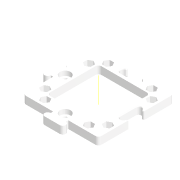
# Autodesk Inventor part: 10_Base_puzzle_v3
Saved by Autodesk Inventor 2022 (Build 260153000, 153)
## iProperties
Created: 2017-06-20
Part Number: 10_Base_puzzle_v3
Material: Generisch
Document SubType Name: Modeling
Designer: diederichbenedict
Density: 1 g/cm^3
Appearance: Weiß
Mass: 5.4697 g
Surface Area: 48.9743 cm^2
Volume: 5.4697 cm^3
Catalog Web Link: isInjectionmolded
Vendor: openUC2
d_part: 50,000 mm
d_o: 40,000 mm
d_i: 40,000 mm
Author: diederichbenedict
Autodesk Inventor part; units mm, degrees
ref_plane "YZ Plane" through (0, 0, 0) normal (1, 0, 0) x (0, 1, 0)
ref_plane "XZ Plane" through (0, 0, 0) normal (0, 1, 0) x (-1, 0, 0)
ref_plane "XY Plane" through (0, 0, 0) normal (0, 0, 1) x (1, 0, 0)
sketch "Skizze1" plane through (0, 0, 0) normal (0, 0, 1) x (1, 0, 0)
  line L0 (-17, 0) -> (-25, 0)
  line L1 (-25, 0) -> (-25, -23)
  line L2 (-23, -25) -> (0, -25)
  line L3 (0, -25) -> (0, -17)
  line L4 (-17, 0) -> (-17, -15)
  line L5 (-15, -17) -> (0, -17)
  arc A0 (-25, -23) -> (-23, -25) centre (-23, -23) ccw
  circle A1 centre (-20.8, -14.5) radius 2.55 construction
  circle A2 centre (-14.5, -20.8) radius 2.55 construction
  arc A3 (-17, -15) -> (-15, -17) centre (-15, -15) ccw
  circle A4 centre (-14.5, -20.8) radius 2.55 construction
  circle A5 centre (-20.8, -14.5) radius 2.55 construction
  line L6 (-30.497056, 0) -> (5.082843, 0) construction
  line L7 (0, -30.497056) -> (0, 5.082843) construction
  line L8 (-18.25, -13.027757) -> (-18.25, -15.972243)
  line L9 (-18.25, -15.972243) -> (-20.8, -17.444486)
  line L10 (-20.8, -17.444486) -> (-23.35, -15.972243)
  line L11 (-23.35, -15.972243) -> (-23.35, -13.027757)
  line L12 (-23.35, -13.027757) -> (-20.8, -11.555514)
  line L13 (-20.8, -11.555514) -> (-18.25, -13.027757)
  line L14 (-15.972243, -18.25) -> (-13.027757, -18.25)
  line L15 (-13.027757, -18.25) -> (-11.555514, -20.8)
  line L16 (-11.555514, -20.8) -> (-13.027757, -23.35)
  line L17 (-13.027757, -23.35) -> (-15.972243, -23.35)
  line L18 (-15.972243, -23.35) -> (-17.444486, -20.8)
  line L19 (-17.444486, -20.8) -> (-15.972243, -18.25)
  point P0 (-25, -25)
  point P1 (-17, -17)
  dimension "d278" = 25
  dimension "d279" = 25
  dimension "d2" = 8
  dimension "d281" = 8
  dimension "d282" = 2
  dimension "d286" = 5.1
  dimension "d_hole" = 5.1
  dimension "d290" = 20.8
  dimension "d" = 20.8
  dimension "d292" = 2
  dimension "d313" = 6.3
  dimension "d314" = 6.3
  dimension "d331" = 0
  dimension "d332" = 0
  constraints: 36 end point, 6 centre point, 6 tangent, 5 coincident, 4 parallel, 4 point on circle, 4 point on line, 2 collinear, 1 horizontal, 1 perpendicular, 26 other
  measures "d278" distance of L2.end point (-25, -25)
  measures "d279" distance of point (-25, -25) L0.end
  measures "d2" distance between parallel lines of L4 L1
  measures "d281" distance between parallel lines of L2 L5
  measures "d282" radius of A0
  measures "d286" diameter of A1
  measures "d_hole" diameter of A2
  measures "d290" distance from line of L0 A2.centre
  measures "d" distance from line of L3 A1.centre
  measures "d292" radius of A3
  measures "d313" horizontal distance of A1.centre A2.centre
  measures "d314" horizontal distance of A1.centre A2.centre
  measures "d331" radial gap between concentric circles of A2 A4
  measures "d332" radial gap between concentric circles of A1 A5
extrude "Extrusion1" add sketch "Skizze1" along normal blind 5
mirror "Mirror6" about plane through (-17, 0, 0) normal (0, 1, 0) of "Extrusion1"
mirror "Mirror7" about plane through (0, -25, 0) normal (1, 0, 0) of "Extrusion1", "Mirror6"
sketch "Sketch26" plane through (0, 0, 5) normal (0, 0, 1) x (1, 0, 0)
  line L0 (23, 25) -> (-23, 25)
  arc A0 (-23, 25) -> (-25, 23) centre (-23, 23) ccw
  line L1 (-25, -23) -> (-25, 23)
  arc A1 (-25, -23) -> (-23, -25) centre (-23, -23) ccw
  line L2 (-23, -25) -> (23, -25)
  arc A2 (23, -25) -> (25, -23) centre (23, -23) ccw
  line L3 (25, 23) -> (25, -23)
  arc A3 (25, 23) -> (23, 25) centre (23, 23) ccw
  line L4 (15, 17) -> (-15, 17)
  arc A4 (17, 15) -> (15, 17) centre (15, 15) ccw
  line L5 (17, 15) -> (17, -15)
  arc A5 (15, -17) -> (17, -15) centre (15, -15) ccw
  line L6 (-15, -17) -> (15, -17)
  arc A6 (-17, -15) -> (-15, -17) centre (-15, -15) ccw
  line L7 (-17, -15) -> (-17, 15)
  arc A7 (-15, 17) -> (-17, 15) centre (-15, 15) ccw
  line L8 (-25, -23) -> (-25, 23)
  line L9 (-28.6, -7) -> (-28.6, -7)
  line L10 (-30.6, -5) -> (-30.6, 5)
  line L11 (-28.6, 7) -> (-28.6, 7)
  line L12 (-25, 16.831111) -> (-25, -7)
  line L13 (-26.363932, 5) -> (-25, 5)
  line L14 (-25, -5) -> (-26.363932, -5)
  arc A8 (-30.6, -5) -> (-28.6, -7) centre (-28.6, -5) ccw
  arc A9 (-28.6, -7) -> (-26.612384, -5.222222) centre (-28.6, -5) ccw
  arc A10 (-28.6, 7) -> (-30.6, 5) centre (-28.6, 5) ccw
  arc A11 (-26.612384, 5.222222) -> (-28.6, 7) centre (-28.6, 5) ccw
  arc A12 (-26.363932, -5) -> (-26.612384, -5.222222) centre (-26.363932, -5.25) ccw
  arc A13 (-26.612384, 5.222222) -> (-26.363932, 5) centre (-26.363932, 5.25) ccw
  line L15 (-42.419899, 0) -> (36.719899, 0)
  point P0 (0, 0)
  point P1 (-24.031265, 1.861044)
  point P2 (-28.6, -7)
  point P3 (-25, -5)
  point P4 (-25, 5)
  point P5 (-28.6, 7)
  dimension "d293" = 5.6
  dimension "d300" = 2
  dimension "d301" = 0.25
  dimension "d365" = 7
  dimension "d367" = 7
  dimension "d385" = 5
  dimension "d386" = 5
  constraints: 12 end point, 12 point on circle, 10 tangent, 6 centre point, 4 equal radius, 3 parallel, 2 coincident, 2 point on line, 1 horizontal, 1 perpendicular, 1 other
  measures "d293" distance between parallel lines of L1 L10
  measures "d300" radius of A8
  measures "d301" radius of A12
  measures "d385" distance of the line from the sketch origin of L14
  measures "d386" distance of the line from the sketch origin of L13
extrude "Extrusion13" add sketch "Sketch26" against normal up to surface (5 mm away) contours L1 L15 L10 A10 A11 A13 L13 | L1 L14 A12 A9 A8 L10 L15
sketch "Sketch28" plane through (0, 0, 5) normal (0, 0, 1) x (1, 0, 0)
  line L0 (-42.039857, 0) -> (37.303501, 0) construction
  line L1 (23, 25) -> (-23, 25)
  arc A0 (-23, 25) -> (-25, 23) centre (-23, 23) ccw
  line L2 (-25, 5) -> (-25, 23)
  arc A1 (-25, -23) -> (-23, -25) centre (-23, -23) ccw
  line L3 (-23, -25) -> (23, -25)
  arc A2 (23, -25) -> (25, -23) centre (23, -23) ccw
  line L4 (25, 23) -> (25, -23)
  arc A3 (25, 23) -> (23, 25) centre (23, 23) ccw
  line L5 (15, 17) -> (-15, 17)
  arc A4 (17, 15) -> (15, 17) centre (15, 15) ccw
  line L6 (17, 15) -> (17, -15)
  arc A5 (15, -17) -> (17, -15) centre (15, -15) ccw
  line L7 (-15, -17) -> (15, -17)
  arc A6 (-17, -15) -> (-15, -17) centre (-15, -15) ccw
  line L8 (-17, -15) -> (-17, 15)
  arc A7 (-15, 17) -> (-17, 15) centre (-15, 15) ccw
  line L9 (24.462448, 5.105821) -> (23.922082, 5.105821) construction
  line L10 (19.183333, 5.062472) -> (23.383333, 5.062472) construction
  line L11 (19.183333, 5.062472) -> (23.383333, 5.062472) construction
  line L12 (23.383333, 5.062472) -> (23.413795, 5.03201) construction
  line L13 (23.383333, 5.062472) -> (23.743079, 5.062472) construction
  line L14 (25, 5) -> (25, 0.105821)
  line L15 (25, 23) -> (25, -23)
  line L16 (24.462448, 5.105821) -> (25, 5.643373) construction
  line L17 (25, 5) -> (25.236865, 5) construction
  line L18 (25, 5.643373) -> (25, 5)
  line L19 (-25, 5) -> (-26.363932, 5) construction
  arc A8 (-26.612384, 5.222222) -> (-26.363932, 5) centre (-26.363932, 5.25) ccw construction
  arc A9 (-26.612384, 5.222222) -> (-30.6, 5) centre (-28.6, 5) ccw construction
  line L20 (-30.6, 5) -> (-30.6, -5) construction
  arc A10 (-30.6, -5) -> (-26.612384, -5.222222) centre (-28.6, -5) ccw construction
  arc A11 (-26.363932, -5) -> (-26.612384, -5.222222) centre (-26.363932, -5.25) ccw construction
  line L21 (-26.363932, -5) -> (-25, -5) construction
  line L22 (-25, -23) -> (-25, -5)
  line L23 (24.462448, -5.105821) -> (23.922082, -5.105821) construction
  line L24 (19.183333, -5.062472) -> (23.383333, -5.062472) construction
  line L25 (19.183333, -5.062472) -> (23.383333, -5.062472) construction
  line L26 (23.383333, -5.062472) -> (23.413795, -5.03201) construction
  line L27 (23.383333, -5.062472) -> (23.743079, -5.062472) construction
  line L28 (25, -5) -> (25, 0.105821)
  line L29 (24.462448, -5.105821) -> (25, -5.643373) construction
  line L30 (25, -5) -> (25.236865, -5) construction
  line L31 (25, -5.643373) -> (25, -5)
  line L32 (21.3, -6.95) -> (21.3, -6.95) construction
  line L33 (19.3, -4.95) -> (19.3, 5.05) construction
  line L34 (21.3, 7.05) -> (21.3, 7.05) construction
  line L35 (23.52262, 5.149812) -> (25, 5.149687) construction
  line L36 (25, -5.050125) -> (23.522632, -5.05) construction
  arc A12 (19.3, -4.95) -> (21.3, -6.95) centre (21.3, -4.95) ccw construction
  arc A13 (21.3, -6.95) -> (23.275654, -5.261111) centre (21.3, -4.95) ccw construction
  arc A14 (21.3, 7.05) -> (19.3, 5.05) centre (21.3, 5.05) ccw construction
  arc A15 (23.275681, 5.360944) -> (21.3, 7.05) centre (21.3, 5.05) ccw construction
  arc A16 (23.522632, -5.05) -> (23.275654, -5.261111) centre (23.522611, -5.3) ccw construction
  arc A17 (23.275681, 5.360944) -> (23.52262, 5.149812) centre (23.522641, 5.399812) ccw construction
  line L37 (-30.6, 5) -> (-30.6, -5)
  line L38 (-25, 5) -> (-26.363932, 5)
  line L39 (-25, 5) -> (-26.363932, 5)
  arc A18 (-26.612384, 5.222222) -> (-26.363932, 5) centre (-26.363932, 5.25) ccw
  arc A19 (-26.612384, 5.222222) -> (-26.363932, 5) centre (-26.363932, 5.25) ccw
  arc A20 (-26.612384, 5.222222) -> (-30.6, 5) centre (-28.6, 5) ccw
  line L40 (-30.6, 5) -> (-30.6, 0)
  line L41 (25, 5.149687) -> (23.467457, 5.149817)
  arc A21 (23.467457, 5.149817) -> (19.55, 5.05) centre (21.51, 5.05) ccw
  line L42 (19.55, 5.05) -> (19.55, 0)
  line L43 (24.462448, -5.105821) -> (23.922082, -5.105821) construction
  line L44 (19.183333, -5.062472) -> (23.383333, -5.062472) construction
  line L45 (19.183333, -5.062472) -> (23.383333, -5.062472) construction
  line L46 (23.383333, -5.062472) -> (23.413795, -5.03201) construction
  line L47 (23.383333, -5.062472) -> (23.743079, -5.062472) construction
  line L48 (25, -5) -> (25, -0.105821)
  line L49 (24.462448, -5.105821) -> (25, -5.643373) construction
  line L50 (25, -5) -> (25.236865, -5) construction
  line L51 (25, -5.643373) -> (25, -5)
  arc A22 (23.52262, -5.149812) -> (23.275681, -5.360944) centre (23.522641, -5.399812) ccw construction
  arc A23 (21.3, -7.05) -> (23.275681, -5.360944) centre (21.3, -5.05) ccw construction
  line L52 (23.52262, -5.149812) -> (25, -5.149687) construction
  arc A24 (19.3, -5.05) -> (21.3, -7.05) centre (21.3, -5.05) ccw construction
  line L53 (25, -5.149687) -> (23.467457, -5.149817)
  arc A25 (19.55, -5.05) -> (23.467457, -5.149817) centre (21.51, -5.05) ccw
  arc A26 (23.467457, -5.149817) -> (23.467457, -5.149817) centre (23.317457, -5.149986) ccw
  line L54 (19.55, -5.05) -> (19.55, 0)
  line L55 (19.55, 0) -> (25, 0)
  point P0 (23.349542, 5.105821)
  point P1 (23.349542, -5.105821)
  point P2 (25, -7)
  point P3 (25.968735, 1.861044)
  point P4 (23.349542, -5.105821)
  point P5 (25.968735, -1.861044)
  point P6 (23.467457, -5.149817)
  dimension "d27" = 0
  dimension "d28" = 0
  dimension "d369" = 4.2
  dimension "d370" = 0
  dimension "d380" = 45
  dimension "d387" = 2
  dimension "d388" = 0.25
  dimension "d391" = 0.1
  dimension "d392" = 5.05
  dimension "d393" = 5.05
  dimension "d394" = 1.96
  dimension "d396" = 5.45
  dimension "d397" = 7.05
  constraints: 80 end point, 30 symmetric about line, 28 point on circle, 14 centre point, 14 tangent, 8 point on line, 5 horizontal, 4 collinear, 4 equal radius, 3 coincident, 2 parallel, 2 perpendicular, 1 midpoint, 4 other
  measures "d369" distance of L10.start L10.end
  measures "d370" distance between parallel lines of L10 L11
  measures "d380" angle of L17 L16
  measures "d387" radius of A12
  measures "d388" radius of A16
  measures "d391" distance from line of L35 A15.centre
  measures "d392" distance from line of L0 A15.centre
  measures "d393" distance from line of L0 A21.centre
  measures "d394" radius of A21
  measures "d396" distance between parallel lines of L4 L42
  measures "d397" distance from line of L0 L34.end
sketch "Sketch28 outline for Extrusion14" plane through (0, 0, 5) normal (0, 0, 1) x (1, 0, 0)
  line L0 (25, 5.149687) -> (23.467457, 5.149817)
  line L1 (25, -5.149687) -> (25, 5.149687)
  line L2 (23.467457, -5.149817) -> (25, -5.149687)
  arc A0 (19.55, -5.05) -> (23.467457, -5.149817) centre (21.51, -5.05) ccw
  line L3 (19.55, 0) -> (19.55, -5.05)
  line L4 (19.55, 5.05) -> (19.55, 0)
  arc A1 (23.467457, 5.149817) -> (19.55, 5.05) centre (21.51, 5.05) ccw
extrude "Extrusion14" cut sketch "Sketch28 outline for Extrusion14" against normal blind 10
pattern_circular "Circular Pattern6" count 2 over 90 about axis through (0, 0, 5) along (0, 0, 1) of "Extrusion14", "Extrusion13"
sketch "Sketch29" plane through (0, 0, 5) normal (0, 0, 1) x (1, 0, 0)
  arc A0 (-23, 25) -> (-25, 23) centre (-23, 23) ccw
  line L0 (-25, 5) -> (-25, 23)
  arc A1 (-25, -23) -> (-23, -25) centre (-23, -23) ccw
  line L1 (-23, -25) -> (-5, -25)
  arc A2 (23, -25) -> (25, -23) centre (23, -23) ccw
  arc A3 (25, 23) -> (23, 25) centre (23, 23) ccw
  line L2 (15, 17) -> (-15, 17)
  arc A4 (17, 15) -> (15, 17) centre (15, 15) ccw
  line L3 (17, 15) -> (17, -15)
  arc A5 (15, -17) -> (17, -15) centre (15, -15) ccw
  line L4 (-15, -17) -> (15, -17)
  arc A6 (-17, -15) -> (-15, -17) centre (-15, -15) ccw
  line L5 (-17, -15) -> (-17, 15)
  arc A7 (-15, 17) -> (-17, 15) centre (-15, 15) ccw
  circle A8 centre (-22, 0) radius 3.89
  circle A9 centre (0, -22) radius 2.925915
  line L6 (-41.928953, 0) -> (36.638075, 0) construction
  line L7 (0, -41.928953) -> (0, 36.638075) construction
  line L8 (25, -5.149687) -> (25, -23)
  line L9 (-5.149687, 25) -> (-23, 25)
  line L10 (-25, 5) -> (-26.363932, 5)
  arc A10 (-26.612384, 5.222222) -> (-26.363932, 5) centre (-26.363932, 5.25) ccw
  arc A11 (-26.612384, 5.222222) -> (-30.6, 5) centre (-28.6, 5) ccw
  line L11 (-30.6, 5) -> (-30.6, -5)
  arc A12 (-30.6, -5) -> (-26.612384, -5.222222) centre (-28.6, -5) ccw
  arc A13 (-26.363932, -5) -> (-26.612384, -5.222222) centre (-26.363932, -5.25) ccw
  line L12 (-26.363932, -5) -> (-25, -5)
  line L13 (-25, -23) -> (-25, -5)
  line L14 (-5, -25) -> (-5, -26.363932)
  arc A14 (-5.222222, -26.612384) -> (-5, -26.363932) centre (-5.25, -26.363932) ccw
  arc A15 (-5.222222, -26.612384) -> (-5, -30.6) centre (-5, -28.6) ccw
  line L15 (-5, -30.6) -> (5, -30.6)
  arc A16 (5, -30.6) -> (5.222222, -26.612384) centre (5, -28.6) ccw
  arc A17 (5, -26.363932) -> (5.222222, -26.612384) centre (5.25, -26.363932) ccw
  line L16 (5, -26.363932) -> (5, -25)
  line L17 (5, -25) -> (23, -25)
  line L18 (-5.149817, 23.467457) -> (-5.149687, 25)
  line L19 (25, -5.149687) -> (23.467457, -5.149817)
  arc A18 (19.55, -5.05) -> (23.467457, -5.149817) centre (21.51, -5.05) ccw
  line L20 (19.55, -5.05) -> (19.55, 5.05)
  arc A19 (23.467457, 5.149817) -> (19.55, 5.05) centre (21.51, 5.05) ccw
  line L21 (23.467457, 5.149817) -> (25, 5.149687)
  line L22 (25, 23) -> (25, 5.149687)
  line L23 (23, 25) -> (5.149687, 25)
  line L24 (5.149687, 25) -> (5.149817, 23.467457)
  arc A20 (5.05, 19.55) -> (5.149817, 23.467457) centre (5.05, 21.51) ccw
  line L25 (5.05, 19.55) -> (-5.05, 19.55)
  arc A21 (-5.149817, 23.467457) -> (-5.05, 19.55) centre (-5.05, 21.51) ccw
  point P0 (0, 0)
  dimension "d319" = 7.78
  dimension "d320" = 5
  dimension "d322" = 5
  constraints: 2 centre point, 2 point on line, 1 coincident
  measures "d319" diameter of A8
  measures "d320" distance from line of A8.centre L5
  measures "d322" distance from line of L4 A9.centre
hole "Hole7" at (-22, 0, 5) at (0, -22, 5) direction (0, 0, -1) diameter 3.2 end through all counterbore diameter 7 counterbore depth 3
chamfer "Fase4" [suppressed]
fillet "Rundung5" radius 0.75 22 edges at (0, 19.55, 5) (-7.0094, 21.4601, 5) (-5.1498, 24.2337, 5) (5.1498, 24.2337, 5) (7.0094, 21.4601, 5) (21.4601, 7.0094, 5) (24.2337, 5.1498, 5) (21.4601, -7.0094, 5) (24.2337, -5.1498, 5) (19.55, 0, 5) (7.0094, 21.4601, 0) (5.1498, 24.2337, 0) (-7.0094, 21.4601, 0) (-5.1498, 24.2337, 0) (0, 19.55, 0) (25, 5.1497, 2.5) (-5.1497, 25, 2.5) (5.1497, 25, 2.5) (-5.1498, 23.4675, 2.5) (5.1498, 23.4675, 2.5) (23.4675, 5.1498, 2.5) (23.4675, -5.1498, 2.5)
equation "\"d27\" = 0"
equation "\"d28\" = 0"
equation "\"d_i\" = 40"
equation "\"d_o\" = 40"
equation "\"d_part\" = 50"
equation "\"d6\" = 0"
equation "\"d7\" = 0"
equation "\"d8\" = 0"
equation "\"d9\" = 0"
equation "\"d13\" = 0"
equation "\"d14\" = 0"
equation "\"d20\" = 0"
equation "\"d21\" = 0"
equation "\"d22\" = 0"
equation "\"d23\" = 0"
equation "\"d24\" = 0"
equation "\"d25\" = 3"
equation "\"d26\" = 0"
equation "\"d29\" = 0"
equation "\"d30\" = 0"
equation "\"d31\" = 0"
equation "\"d32\" = 0"
equation "\"d33\" = 0"
equation "\"d34\" = 0"
equation "\"d46\" = 0"
equation "\"d47\" = 0"
equation "\"d48\" = 0"
equation "\"d50\" = 0"
equation "\"d51\" = 0"
equation "\"d52\" = 0"
equation "\"d53\" = 0"
equation "\"d54\" = 0"
equation "\"d55\" = 0"
equation "\"d56\" = 0"
equation "\"d57\" = 0"
equation "\"d58\" = 0"
equation "\"d59\" = 0"
equation "\"magnet_offset\" = 0"
equation "\"screw_offset\" = 0"
equation "\"mal_puzzle_offset\" = 0"
equation "\"fem_puzzle_offset\" = 0"
